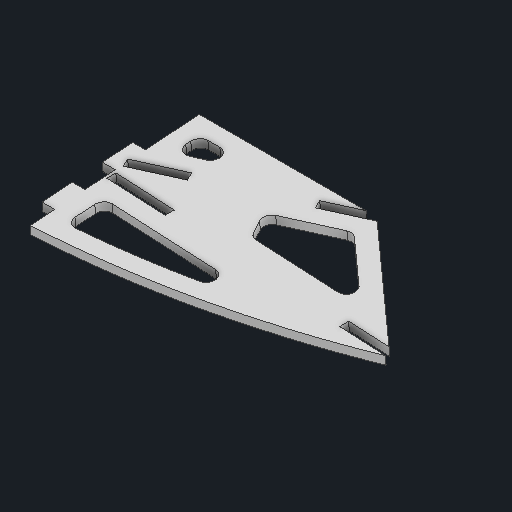
# Autodesk Inventor part: sponson_break
Saved by Autodesk Inventor 2023 (Build 270158030, 158C)
## iProperties
Created: 2022-03-21
Part Number: sponson_break
Material: Generic
Document SubType Name: Modeling
Designer: kardo
Density: 1 g/cm^3
Appearance: Default
Author: kardo
Autodesk Inventor part; units mm, degrees
ref_plane "YZ Plane" through (0, 0, 0) normal (1, 0, 0) x (0, 1, 0)
ref_plane "XZ Plane" through (0, 0, 0) normal (0, 1, 0) x (-1, 0, 0)
ref_plane "XY Plane" through (0, 0, 0) normal (0, 0, 1) x (1, 0, 0)
derived "parameters_frame.ipt"
derived "surface_body.ipt"
sketch "sk_rail_sponson_tunnel" plane through (81.12, 0, 0) normal (1, 0, 0) x (0, 1, 0)
  line L0 (0, 0) -> (122.4, 8.559)
  line L1 (112.6461, 148.0459) -> (139.8617, -241.1549) construction
  spline S0 degree 2 poles (122.4, 8.559) (190.3044, 13.3074) (255, 36.448) knots 0 0 0 1 1 1
sketch "sk_rail_sponson_bottom" plane through (126.048, 0, 0) normal (0.3820078, -0.0644661, 0.9219079) x (-0.1718217, 0.9752166, 0.139391)
  line L0 (120.5596, -22.8124) -> (0, 0)
  line L1 (389.238, -73.6522) -> (-473.5511, 89.606) construction
  line L2 (163.9663, 206.5842) -> (90.6689, -180.7791) construction
  spline S0 degree 2 poles (120.5596, -22.8124) (192.7887, -36.4798) (261.4804, 0) knots 0 0 0 1 1 1
  point P0 (21.6578, 114.4574)
sketch "sk_rail_sponson_side" plane through (81.12, 255, 36.448) normal (0.0461938, 0.0348622, -0.998324) x (0.2816917, -0.9592867, -0.0204648)
  line L0 (265.8225, 0) -> (150.1079, -34.011)
  spline S0 degree 2 poles (150.1079, -34.011) (71.6005, -57.0859) (0, 0) knots 0 0 0 1 1 1
  point P0 (222.5132, 151.1878)
ref_plane "plane_sponson_break" through (0, 122.4, 8.559) normal (0, 0.9975641, 0.0697565) x (-1, 0, 0)
sketch "sk_section_sponson_break" plane through (0, 122.4, 8.559) normal (0, 0.9975641, 0.0697565) x (-1, 0, 0)
  line L0 (-273.529, -60.9623) -> (62.2867, 77.8495) construction
  line L1 (-81.12, -262.9814) -> (-81.12, 151.9167) construction
  arc A0 (-81.12, 42.1186) -> (-156, 26.7233) centre (-71.3066, -195.4114) ccw construction
  arc A1 (-54.6, 54.2675) -> (-156, 30.9325) centre (-53.2768, -183.4615) ccw construction
  spline S0 degree 2 poles (-54.6, 54.2675) (-107.2974, 54.2675) (-156, 30.9325) knots 0 0 0 1 1 1
  spline S1 degree 2 poles (-156, 26.7233) (-120.0524, 40.429) (-81.12, 42.1186) knots 0 0 0 1 1 1
  point P0 (0, 0)
derived "stencil_frame.ipt"
sketch "sk_joint_locations" plane through (81.12, 0, 0) normal (1, 0, 0) x (0, 1, 0)
  line L0 (0, 0) -> (122.4, 8.559) construction
  line L1 (36.465, 28.832) -> (112.2, 28.832) construction
  arc A0 (36.465, 28.832) -> (11.22, 28.376) centre (36.465, -670.197) ccw construction
  line L2 (-241.5001, 19.2432) -> (11.22, 28.376) construction
  line L3 (-345, 16.32) -> (-262.2001, 18.586) construction
  arc A1 (-262.2001, 18.586) -> (-241.5001, 19.2432) centre (-326.8578, 2381.2399) ccw construction
  line L4 (-95.1358, 3119.4657) -> (254.2444, -1876.9042) construction
  line L5 (-230.0001, 3089.1136) -> (-230.0001, -1866.0023) construction
  line L6 (-114.9999, 3089.1136) -> (-114.9999, -1866.0023) construction
  line L7 (-345, 3089.1136) -> (-345, -1866.0023) construction
  line L8 (0, 3089.1136) -> (0, -1866.0023) construction
  line L9 (516.4305, 45.5774) -> (-594.5903, 6.7797) construction
  line L10 (-657.7604, -27.3784) -> (621.8174, 62.0984) construction
  line L11 (193.4506, 30.2962) -> (193.1714, 38.2913) construction
  line L12 (201.1621, 36.7028) -> (201.7215, 28.7028) construction
  line L13 (0, 14.96) -> (121.9304, 15.2746) construction
  line L14 (-230.0001, 45.8702) -> (-230.0001, 19.6588) construction
  line L15 (-345, 37.4554) -> (-345, 16.32) construction
  line L16 (-114.9999, 51.0173) -> (-114.9999, 23.8147) construction
  line L17 (0, 52.89) -> (0, 27.9705) construction
  line L18 (119.462, 50.575) -> (119.9556, 43.5149) construction
  line L19 (120.4493, 36.4549) -> (119.9556, 43.5149) construction
  line L20 (120.4493, 36.4549) -> (120.943, 29.3948) construction
  line L21 (120.943, 29.3948) -> (121.4367, 22.3347) construction
  line L22 (121.4367, 22.3347) -> (121.9304, 15.2746) construction
  line L23 (0, 14.96) -> (0, 0) construction
  spline S0 degree 4 poles (-345, 37.4554) (-258.8682, 45.1562) (-172.5926, 49.7838) (-86.3161, 52.89) (0, 52.89) knots 0 0 0 0 0 1 1 1 1 1
  spline S1 degree 3 poles (0, 52.89) (92.8353, 52.89) (195.0311, 49.5089) (255, 36.448) knots 0 0 0 0 1 1 1 1
  spline S2 degree 2 poles (122.4, 8.559) (190.3044, 13.3074) (255, 36.448) knots 0 0 0 1 1 1
  line L24 (112.2, 37.536) -> (112.2, 28.832) construction
  line L25 (112.2, 35.548) -> (112.2, 30.82) construction
  point P0 (-95.1358, 3119.4657)
  point P1 (254.2444, -1876.9042)
  point P2 (193.311, 34.2938)
  point P3 (201.4418, 32.7028)
  point P4 (134.9575, 11.3411)
  point P5 (-345, 26.8877)
  point P6 (-230.0001, 32.7645)
  point P7 (-114.9999, 37.416)
  point P8 (0, 40.4303)
  point P9 (112.2, 33.184)
sketch "sk_spanner_joints_locations" plane through (0, 122.4, 8.559) normal (0, 0.9975641, 0.0697565) x (-1, 0, 0)
  line L0 (300.9234, 5.5808) -> (-420.7494, 38.9736) construction
  line L1 (-923.3057, -329.5522) -> (1264.6454, 574.8532) construction
  line L2 (-84.7099, 23.4246) -> (-83.6779, 17.514) construction
  line L3 (-84.7099, 23.4246) -> (-70.9223, 22.7866) construction
  line L4 (-83.6779, 17.514) -> (-70.9223, 22.7866) construction
  point P0 (0, 0)
  point P1 (-126.048, 0)
  point P2 (-156, 26.7233)
  point P3 (-141.742, 26.0635)
  point P4 (-98.9679, 24.0843)
  point P5 (-94.2704, 13.1355)
  point P6 (-115.4555, 4.3785)
sketch "sk_sponson_break_base" plane through (0, 122.4, 8.559) normal (0, 0.9975641, 0.0697565) x (-1, 0, 0)
  spline S0 degree 2 poles (-156, 26.7233) (-120.0524, 40.429) (-81.12, 42.1186) knots 0 0 0 1 1 1 construction
  line L0 (-156, 26.7233) -> (-126.048, 0) construction
  line L1 (-126.048, 0) -> (-81.12, 0) construction
  line L2 (-81.12, 35.0412) -> (-81.12, 27.9639)
  line L3 (-81.12, 27.9639) -> (-84.12, 27.9639)
  line L4 (-81.12, 35.0412) -> (-84.12, 35.0412)
  line L5 (-84.12, 35.0412) -> (-84.12, 40.7684)
  line L6 (-84.12, 27.9639) -> (-84.12, 20.8866)
  line L7 (-84.12, 20.8866) -> (-81.12, 20.8866)
  line L8 (-81.12, 20.8866) -> (-81.12, 13.8093)
  line L9 (-81.12, 13.8093) -> (-84.12, 13.8093)
  line L10 (-84.12, 13.8093) -> (-84.12, 1.2)
  line L11 (-153.7218, 26.2989) -> (-125.5905, 1.2)
  line L12 (-125.5905, 1.2) -> (-84.12, 1.2)
  spline S1 degree 5 poles (-84.12, 40.7684) (-98.3699, 39.9741) (-112.5625, 38.1523) (-126.5961, 35.2489) (-140.3446, 31.2729) (-153.7218, 26.2988) knots 0 0 0 0 0 0 1 1 1 1 1 1
  point P0 (0, 0)
  point P1 (-156, 26.7233)
  dimension "d4" = 1.2
  dimension "d3" = 3
  constraints: 26 end point, 6 parallel, 4 perpendicular, 1 vertical, 4 other
  measures "d3" distance from line of L7.end L6
extrude "thicken" add sketch "sk_sponson_break_base" against normal blind 2
sketch "sk_spanner_joints" plane through (0, 122.4, 8.559) normal (0, 0.9975641, 0.0697565) x (-1, 0, 0)
  line L0 (-156, 26.7233) -> (-141.742, 26.0635)
  line L1 (-141.742, 26.0635) -> (-141.8344, 24.0657)
  line L2 (-141.8344, 24.0657) -> (-156.0924, 24.7254)
  line L3 (-156.0924, 24.7254) -> (-156, 26.7233)
  line L4 (-98.9679, 24.0843) -> (-99.0604, 22.0864)
  line L5 (-99.0604, 22.0864) -> (-84.8023, 21.4267)
  line L6 (-84.8023, 21.4267) -> (-84.7099, 23.4246)
  line L7 (-98.9679, 24.0843) -> (-84.7099, 23.4246)
  line L8 (-94.2704, 13.1355) -> (-95.0344, 14.9838)
  line L9 (-95.0344, 14.9838) -> (-84.4419, 19.3623)
  line L10 (-84.4419, 19.3623) -> (-83.6779, 17.514)
  line L11 (-83.6779, 17.514) -> (-94.2704, 13.1355)
  line L12 (-126.048, 0) -> (-115.4555, 4.3785)
  line L13 (-115.4555, 4.3785) -> (-116.2195, 6.2268)
  line L14 (-116.2195, 6.2268) -> (-126.812, 1.8483)
  line L15 (-126.812, 1.8483) -> (-126.048, 0)
  point P0 (0, 0)
  dimension "d7" = 2
  constraints: 32 end point, 8 perpendicular, 7 equal length
  measures "d7" distance of L2.end L0.start
extrude "cut_spanner_joints" cut sketch "sk_spanner_joints" along normal through all both and the other way through all
sketch "sk_cut_weight" plane through (0, 122.4, 8.559) normal (0, 0.9975641, 0.0697565) x (-1, 0, 0)
  spline S0 degree 3 poles (-84.12, 40.7684) (-88.1317, 40.5448) (-95.1097, 39.9842) (-102.9997, 39.0051) (-108.8809, 38.1257) (-112.7836, 37.4669) (-117.6394, 36.5528) (-121.5059, 35.7489) (-126.3165, 34.6535) (-130.147, 33.7046) (-134.9125, 32.4278) (-138.707, 31.3338) (-143.4276, 29.8757) (-148.1258, 28.3268) (-151.8605, 26.991) (-153.7218, 26.2989) knots 0.025843 0.025843 0.025843 0.025843 0.181628 0.298467 0.337413 0.415306 0.454252 0.532145 0.571091 0.648984 0.68793 0.765823 0.804769 0.882662 0.960554 0.960554 0.960554 0.960554 construction
  line L0 (-153.7218, 26.2989) -> (-125.5905, 1.2) construction
  line L1 (-125.5905, 1.2) -> (-84.12, 1.2) construction
  line L2 (-84.7099, 23.4246) -> (-156, 26.7233) construction
  line L3 (-83.6779, 17.514) -> (-126.048, 0) construction
  line L4 (-79.9867, 21.2039) -> (-151.7321, 24.5236) construction
  line L5 (-79.9867, 21.2039) -> (-126.4738, 1.9881) construction
  line L6 (-84.12, 40.7684) -> (-84.12, 1.2) construction
  line L7 (-88.12, 36.5023) -> (-88.12, 27.5866)
  line L8 (-88.12, 27.5866) -> (-130.2323, 29.5352)
  line L9 (-104.8552, 1.2) -> (-115.8594, 22.8638) construction
  line L10 (-140.6616, 20.0071) -> (-113.7765, 18.7631)
  line L11 (-110.7546, 12.814) -> (-125.6831, 6.6432)
  line L12 (-125.6831, 6.6432) -> (-140.6616, 20.0071)
  line L13 (-113.7765, 18.7631) -> (-110.7546, 12.814)
  line L14 (-88.12, 11.3496) -> (-102.9971, 5.2)
  line L15 (-102.9971, 5.2) -> (-88.12, 5.2)
  line L16 (-88.12, 5.2) -> (-88.12, 11.3496)
  spline S1 degree 4 poles (-88.12, 36.5023) (-98.7774, 35.7211) (-109.3902, 34.31) (-119.8947, 32.2422) (-130.2322, 29.5352) knots 0 0 0 0 0 1 1 1 1 1
  point P0 (0, 0)
  dimension "d12" = 4
  dimension "d10" = 2
  dimension "d11" = 2
  dimension "d13" = 4
  dimension "d14" = 4
  dimension "d15" = 4
  dimension "d16" = 4
  dimension "d17" = 4
  dimension "d18" = 4
  dimension "d19" = 4
  dimension "d20" = 4
  constraints: 30 end point, 10 parallel, 4 point on line, 2 midpoint, 3 other
  measures "d10" distance between parallel lines of L2 L4
  measures "d11" distance between parallel lines of L3 L5
  measures "d13" distance between parallel lines of L2 L8
  measures "d14" distance between parallel lines of L6 L7
  measures "d15" distance between parallel lines of L0 L12
  measures "d16" distance between parallel lines of L4 L10
  measures "d17" distance between parallel lines of L5 L11
  measures "d18" distance between parallel lines of L1 L15
  measures "d19" distance between parallel lines of L6 L16
  measures "d20" distance between parallel lines of L3 L14
extrude "cut_weight" cut sketch "sk_cut_weight" along normal through all both and the other way through all
fillet "Fillet1" radius 2 10 edges at (102.9971, 121.0397, 13.6766) (88.12, 120.6107, 19.8112) (88.12, 121.0397, 13.6766) (125.6831, 120.939, 15.1163) (110.7546, 120.5086, 21.2721) (88.12, 119.4781, 36.0087) (113.7765, 120.0936, 27.2067) (140.6616, 120.0068, 28.4477) (130.2322, 119.3422, 37.9525) (88.12, 118.8562, 44.9026)
equation "\"d4\" = shell_thickness"
equation "\"d3\" = stringer_thickness"
equation "\"d5\" = bulkhead_thickness"
equation "\"d7\" = bulkhead_thickness"
equation "\"d12\" = bulkhead_inset"
equation "\"d10\" = bulkhead_thickness"
equation "\"d11\" = bulkhead_thickness"
equation "\"d13\" = bulkhead_inset"
equation "\"d14\" = bulkhead_inset"
equation "\"d15\" = bulkhead_inset"
equation "\"d16\" = bulkhead_inset"
equation "\"d17\" = bulkhead_inset"
equation "\"d18\" = bulkhead_inset"
equation "\"d19\" = bulkhead_inset"
equation "\"d20\" = bulkhead_inset"
equation "\"d23\" = 0.5 * bulkhead_inset"
equation "\"shell_thickness\" = 1.2"
equation "\"stringer_thickness\" = 3"
equation "\"bulkhead_thickness\" = 2"
equation "\"bulkhead_inset\" = 4"
body "Solid1"
